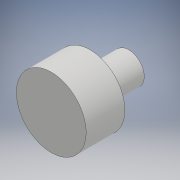
# Autodesk Inventor part: Platform Pin
Saved by Autodesk Inventor 2017 (Build 210142000, 142)
## iProperties
Created: 2018-03-19
Part Number: Platform Pin
Material: Generic
Document SubType Name: Modeling
Designer: Arjuna
Density: 1 g/cm^3
Appearance: Default
Author: Arjuna
## iProperties of the stored document Platform Pin_3DPrint.ipt
Created: 2018-03-30
Part Number: Platform Pin_3DPrint
Material: Generic
Document SubType Name: Modeling
Designer: Arjuna
Density: 1 g/cm^3
Appearance: Default
Author: Arjuna
Autodesk Inventor part; units mm, degrees
ref_plane "YZ Plane" through (0, 0, 0) normal (1, 0, 0) x (0, 1, 0)
ref_plane "XZ Plane" through (0, 0, 0) normal (0, 1, 0) x (-1, 0, 0)
ref_plane "XY Plane" through (0, 0, 0) normal (0, 0, 1) x (1, 0, 0)
sketch "Sketch1" plane through (0, 0, 0) normal (0, 1, 0) x (-1, 0, 0)
  circle A0 centre (0, 0) radius 4.5
  dimension "d0" = 9
  constraints: 1 centre point, 1 coincident
  measures "d0" diameter of A0
extrude "Extrusion1" add sketch "Sketch1" along normal blind 5
sketch "Sketch2" plane through (0, 5, 0) normal (0, 1, 0) x (1, 0, 0)
  circle A0 centre (0, 0) radius 2
  dimension "d3" = 4
  constraints: 1 centre point, 1 coincident
  measures "d3" diameter of A0
extrude "Extrusion2" add sketch "Sketch2" along normal blind 5
body "Solid1"
